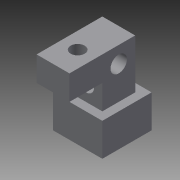
# Autodesk Inventor part: quad
Saved by Autodesk Inventor 2013 (Build 170138000, 138)
## iProperties
Created: 2013-01-16
Part Number: quad
Material: Generic
Document SubType Name: Modeling
Designer: geohot
Density: 1 g/cm^3
Author: geohot
Autodesk Inventor part; units mm, degrees
ref_plane "YZ Plane" through (0, 0, 0) normal (1, 0, 0) x (0, 1, 0)
ref_plane "XZ Plane" through (0, 0, 0) normal (0, 1, 0) x (-1, 0, 0)
ref_plane "XY Plane" through (0, 0, 0) normal (0, 0, 1) x (1, 0, 0)
sketch "Sketch1" plane through (0, 0, 0) normal (0, 0, 1) x (1, 0, 0)
  circle A0 centre (0, 0) radius 1.5875
  line L0 (-3.175, -3.175) -> (3.175, -3.175)
  line L1 (3.175, -3.175) -> (3.175, 6.35)
  line L2 (3.175, 6.35) -> (-3.175, 6.35)
  line L3 (-3.175, 6.35) -> (-3.175, -3.175)
  dimension "d0" = 3.175
  dimension "d2" = 6.35
  dimension "d3" = 3.175
  dimension "d4" = 3.175
  dimension "d5" = 9.525
  constraints: 8 end point, 2 parallel, 1 centre point, 1 coincident, 1 horizontal, 1 perpendicular
  measures "d0" diameter of A0
  measures "d2" distance of L0.start L0.end
  measures "d3" horizontal distance of L0.end point (0, 0)
  measures "d4" distance from line of L0 point (0, 0)
  measures "d5" distance of L0.end L1.end
extrude "Extrusion1" add sketch "Sketch1" along normal blind 6.35
sketch "Sketch2" plane through (3.175, -3.175, 0) normal (1, 0, 0) x (0, 0, -1)
  line L0 (0, 9.525) -> (-6.35, 9.525) projected
  circle A0 centre (-3.175, 6.35) radius 1.5875
  point P0 (0, 3.175)
  dimension "d8" = 3.175
  dimension "d9" = 3.175
  constraints: 1 centre point
  measures "d8" distance from line of L0 A0.centre
  measures "d9" diameter of A0
extrude "Extrusion2" cut sketch "Sketch2" against normal up to next
sketch "Sketch3" plane through (0, 0, 6.35) normal (0, 0, 1) x (1, 0, 0)
  line L0 (3.175, -3.175) -> (3.175, 6.35) projected
  line L1 (-3.175, 6.35) -> (3.175, 6.35)
  line L2 (3.175, 6.35) -> (3.175, 1.5875)
  line L3 (3.175, 1.5875) -> (-3.175, 1.5875)
  line L4 (-3.175, 1.5875) -> (-3.175, 6.35)
  point P0 (3.175, 0)
  constraints: 8 end point, 2 parallel, 1 horizontal, 1 midpoint, 1 perpendicular
extrude "Extrusion3" add sketch "Sketch3" along normal blind 6.35
sketch "Sketch4" plane through (-3.175, 6.35, 0) normal (0, 1, 0) x (1, 0, 0)
  circle A0 centre (3.175, -7.9375) radius 1.3525
  line L0 (6.35, 0) -> (0, 0) projected
  point P0 (3.175, 0)
  dimension "d15" = 2.7051
  dimension "d26" = 7.9375
  constraints: 1 centre point
  measures "d15" diameter of A0
  measures "d26" distance from line of L0 A0.centre
extrude "Extrusion4" cut sketch "Sketch4" against normal blind 6.35
sketch "Sketch5" plane through (-3.175, -3.175, 0) normal (0, -1, 0) x (1, 0, 0)
  line L0 (0, 0) -> (6.35, 0) projected
  line L1 (6.35, 0) -> (6.35, 6.35) projected
  line L2 (0, 6.35) -> (6.35, 6.35) projected
  line L3 (0, 0) -> (0, 6.35) projected
  line L4 (-1.5875, 7.9375) -> (7.9375, 7.9375)
  line L5 (7.9375, 7.9375) -> (7.9375, -1.5875)
  line L6 (7.9375, -1.5875) -> (-1.5875, -1.5875)
  line L7 (-1.5875, -1.5875) -> (-1.5875, 7.9375)
  point P0 (3.175, 0)
  dimension "d20" = 1.5875
  dimension "d21" = 1.5875
  dimension "d22" = 1.5875
  dimension "d23" = 1.5875
  constraints: 8 end point, 2 parallel, 1 horizontal, 1 perpendicular
  measures "d20" distance between parallel lines of L4 L2
  measures "d21" distance between parallel lines of L5 L1
  measures "d22" distance between parallel lines of L6 L0
  measures "d23" distance between parallel lines of L7 L3
extrude "Extrusion5" add sketch "Sketch5" along normal blind 6.35 contours L3 L2 L1 L0 | L4 L5 L6 L7
body "Solid1"
